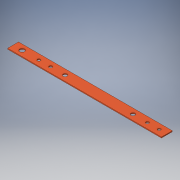
# Autodesk Inventor part: CU6
Saved by Autodesk Inventor 2016 (Build 200138000, 138)
## iProperties
Created: 2018-05-02
Part Number: CU6
Material: Copper
Document SubType Name: Modeling
Designer: Phil Erle
Density: 8.94 g/cm^3
Appearance: Copper - Satin
Author: Phil Erle
Autodesk Inventor part; units mm, degrees
ref_plane "YZ Plane" through (0, 0, 0) normal (1, 0, 0) x (0, 1, 0)
ref_plane "XZ Plane" through (0, 0, 0) normal (0, 1, 0) x (-1, 0, 0)
ref_plane "XY Plane" through (0, 0, 0) normal (0, 0, 1) x (1, 0, 0)
sketch "Sketch1" plane through (0, 0, 0) normal (0, 0, 1) x (1, 0, 0)
  line L0 (-75, -6) -> (75, -6)
  line L1 (75, -6) -> (75, 6)
  line L2 (75, 6) -> (-75, 6)
  line L3 (-75, 6) -> (-75, -6)
  line L4 (-75, -6) -> (75, 6) construction
  line L5 (75, -6) -> (-75, 6) construction
  point P0 (0, 0)
  dimension "d0" = 150
  dimension "d1" = 12
  constraints: 12 end point, 2 midpoint, 2 parallel, 1 horizontal, 1 perpendicular
  measures "d0" distance of L1.end L2.end
  measures "d1" distance of L0.end L1.end
extrude "Extrusion1" add sketch "Sketch1" along normal blind 1
sketch "Sketch2" plane through (0, 0, 1) normal (0, 0, 1) x (1, 0, 0)
  line L0 (-66.5, 0) -> (-53.5, 0) construction
  line L1 (-53.5, 0) -> (53.5, 0) construction
  line L2 (53.5, 0) -> (66.5, 0) construction
  point P0 (0, 0)
  point P1 (0, 0)
  dimension "d4" = 133
  dimension "d5" = 13
  dimension "d6" = 13
  constraints: 6 end point, 5 coincident, 2 point on line, 1 horizontal, 1 horizontal alignment, 1 midpoint
  measures "d4" distance of L2.end L0.start
  measures "d5" distance of L0.start L0.end
  measures "d6" distance of L1.end L2.end
hole "Hole1" at (-66.5, 0, 1) at (-53.5, 0, 1) at (66.5, 0, 1) at (53.5, 0, 1) direction (0, 0, -1) diameter 3.4 depth 8 tip angle 118 clearance for "Countersunk Flat Head Screw DIN EN ISO 2009" size "M3" standard "DIN"
sketch "Sketch4" plane through (0, 0, 1) normal (0, 0, 1) x (1, 0, 0)
  line L0 (-37.5, 0) -> (37.5, 0) construction
  point P0 (0, 0)
  point P1 (0, 0)
  dimension "d21" = 75
  constraints: 3 coincident, 2 end point, 1 horizontal, 1 horizontal alignment, 1 midpoint
  measures "d21" distance of L0.start L0.end
hole "Hole3" at (-37.5, 0, 1) at (37.5, 0, 1) direction (0, 0, -1) diameter 4.5 depth 8 tip angle 118 clearance for "Countersunk Flat Head Screw DIN EN ISO 2009" size "M4" standard "DIN"
sketch "Sketch6" plane through (-75, -6, 0) normal (-1, 0, 0) x (0, 0, 1)
  line L0 (1, 0) -> (1, 12) projected
  line L1 (0, 0) -> (1, 0)
  line L2 (1, 0) -> (1, 12)
  line L3 (1, 12) -> (0, 12)
  line L4 (0, 12) -> (0, 0)
  point P0 (0, 6)
  constraints: 8 end point, 2 coincident, 2 parallel, 1 horizontal, 1 perpendicular
extrude "Extrusion2" add sketch "Sketch6" along normal blind 20
sketch "Sketch7" plane through (0, 0, 1) normal (0, 0, 1) x (1, 0, 0)
  line L0 (-95, -6) -> (-95, 6) projected
  point P0 (0, 0)
  point P1 (-85, 0)
  dimension "d39" = 10
  constraints: 1 horizontal alignment
  measures "d39" distance from line of L0 point (-85, 0)
hole "Hole5" at (-85, 0, 1) direction (0, 0, -1) diameter 5.5 depth 8 tip angle 118 clearance for "Countersunk Flat Head Screw DIN EN ISO 2009" size "M5" standard "DIN"
body "Solid1"
